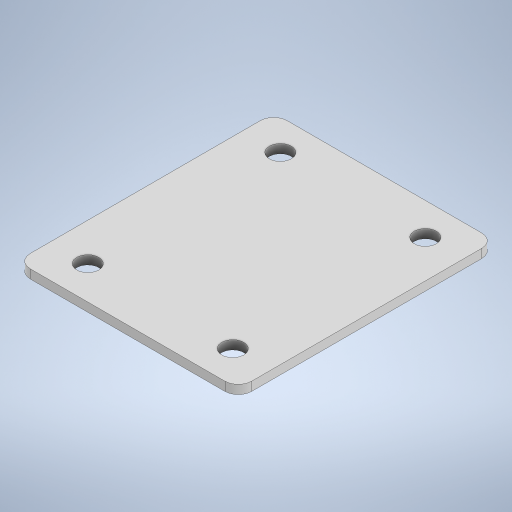
# Autodesk Inventor part: PCB_design
Saved by Autodesk Inventor 2024.2 (Build 282272000, 272)
## iProperties
Created: 2024-04-01
Part Number: PCB_design
Material: Generic
Document SubType Name: Modeling
Designer: ringl
Density: 1 g/cm^3
Appearance: Default
Author: ringl
Autodesk Inventor part; units mm, degrees
ref_plane "YZ Plane" through (0, 0, 0) normal (1, 0, 0) x (0, 1, 0)
ref_plane "XZ Plane" through (0, 0, 0) normal (0, 1, 0) x (-1, 0, 0)
ref_plane "XY Plane" through (0, 0, 0) normal (0, 0, 1) x (1, 0, 0)
sketch "Sketch1" plane through (0, 0, 0) normal (0, 1, 0) x (-1, 0, 0)
  line L0 (0, 0) -> (50, 0)
  line L1 (50, 0) -> (50, -58)
  line L2 (50, -58) -> (0, -58)
  line L3 (0, -58) -> (0, 0)
  circle A0 centre (41.4991, -7.5) radius 2.5
  circle A1 centre (41.4991, -51) radius 2.5
  circle A2 centre (8.5, -50.75) radius 2.5
  circle A3 centre (8.5, -7.25) radius 2.5
  dimension "d0" = 50
  dimension "d1" = 58
  dimension "d2" = 5
  dimension "d3" = 5
  dimension "d4" = 5
  dimension "d5" = 5
  dimension "d7" = 8.5
  dimension "d8" = 33
  dimension "d9" = 33
  dimension "d10" = 7.25
  dimension "d11" = 7
  dimension "d14" = 43.5
  dimension "d15" = 43.5
  constraints: 8 end point, 4 centre point, 2 parallel, 1 horizontal, 1 perpendicular, 1 vertical alignment
  measures "d0" distance of L1.end L2.end
  measures "d1" distance of L0.end L1.end
  measures "d2" diameter of A0
  measures "d3" diameter of A1
  measures "d4" diameter of A2
  measures "d5" diameter of A3
  measures "d7" distance from line of L3 A3.centre
  measures "d8" distance of A2.centre A1.centre
  measures "d9" distance of A0.centre A3.centre
  measures "d10" distance from line of L2 A2.centre
  measures "d11" distance from line of L2 A1.centre
  measures "d14" distance of A1.centre A0.centre
  measures "d15" distance of A2.centre A3.centre
extrude "Extrusion1" add sketch "Sketch1" along normal blind 2
fillet "Fillet1" radius 3 4 edges at (-50, 1, -58) (0, 1, -58) (0, 1, 0) (-50, 1, 0)
body "Solid1"
